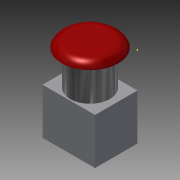
# Autodesk Inventor part: Button
Saved by Autodesk Inventor 2014 SP1 (Build 180222100, 222)
## iProperties
Created: 2014-11-19
Part Number: Button
Material: Generic
Document SubType Name: Modeling
Designer: AlecShufelt
Density: 1 g/cm^3
Appearance: Default
Author: AlecShufelt
Autodesk Inventor part; units mm, degrees
ref_plane "YZ Plane" through (0, 0, 0) normal (1, 0, 0) x (0, 1, 0)
ref_plane "XZ Plane" through (0, 0, 0) normal (0, 1, 0) x (-1, 0, 0)
ref_plane "XY Plane" through (0, 0, 0) normal (0, 0, 1) x (1, 0, 0)
sketch "Sketch1" plane through (0, 0, 0) normal (0, 1, 0) x (-1, 0, 0)
  line L0 (0, 0) -> (36.957, 0)
  line L1 (36.957, 0) -> (36.957, 29.8958)
  line L2 (36.957, 29.8958) -> (0, 29.8958)
  line L3 (0, 29.8958) -> (0, 0)
  dimension "d0" = 36.957
  dimension "d1" = 29.8958
  constraints: 8 end point, 2 parallel, 1 horizontal, 1 perpendicular
  measures "d0" distance of L2.end L1.end
  measures "d1" distance of L0.end L1.end
extrude "Extrusion1" add sketch "Sketch1" along normal blind 32.3596
sketch "Sketch2" plane through (0, 32.3596, 0) normal (0, 1, 0) x (1, 0, 0)
  circle A0 centre (-18.4785, -14.9479) radius 13.97
  dimension "d4" = 27.94
  constraints: 1 centre point
  measures "d4" diameter of A0
extrude "Extrusion2" add sketch "Sketch2" along normal blind 24.6634
sketch "Sketch3" plane through (-18.4785, 57.023, 14.9479) normal (0, 1, 0) x (1, 0, 0)
  circle A0 centre (0, 0) radius 13.97 projected
  point P0 (18.4785, 14.9479)
sketch "Sketch4" plane through (-18.4785, 57.023, 14.9479) normal (0, 1, 0) x (1, 0, 0)
  circle A0 centre (0, 0) radius 13.97 projected
  circle A1 centre (0, 0) radius 19.8628
  point P0 (18.4785, 14.9479)
  dimension "d7" = 39.7256
  constraints: 1 centre point, 1 coincident
  measures "d7" diameter of A1
extrude "Extrusion3" add sketch "Sketch4" along normal blind 4.7498 contours A0 | A1
fillet "Fillet1" radius 7.62 1 edges at (-38.3413, 61.7728, 14.9479)
body "Solid1"
